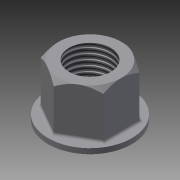
# Autodesk Inventor part: 13_17
Saved by Autodesk Inventor 2015 (Build 190159000, 159)
## iProperties
Created: 2015-04-06
Part Number: 13_17
Material: Generic
Document SubType Name: Modeling
Designer: WASHHSST
Density: 1 g/cm^3
Appearance: Default
Author: WASHHSST
Autodesk Inventor part; units mm, degrees
ref_plane "YZ Plane" through (0, 0, 0) normal (1, 0, 0) x (0, 1, 0)
ref_plane "XZ Plane" through (0, 0, 0) normal (0, 1, 0) x (-1, 0, 0)
ref_plane "XY Plane" through (0, 0, 0) normal (0, 0, 1) x (1, 0, 0)
sketch "Sketch1" plane through (0, 0, 0) normal (0, 1, 0) x (-1, 0, 0)
  circle A0 centre (0, 0) radius 25.4
  dimension "d0" = 50.8
  constraints: 1 centre point, 1 coincident
  measures "d0" diameter of A0
extrude "Extrusion1" add sketch "Sketch1" along normal blind 3.175
sketch "Sketch2" plane through (0, 3.175, 0) normal (0, 1, 0) x (1, 0, 0)
  circle A0 centre (0, 0) radius 19.05
  line L0 (-19.05, -10.9985) -> (-19.05, 10.9985)
  line L1 (-19.05, 10.9985) -> (0, 21.997)
  line L2 (0, 21.997) -> (19.05, 10.9985)
  line L3 (19.05, 10.9985) -> (19.05, -10.9985)
  line L4 (19.05, -10.9985) -> (0, -21.997)
  line L5 (0, -21.997) -> (-19.05, -10.9985)
  point P0 (-9.525, -16.4978)
  dimension "d3" = 38.1
  constraints: 12 end point, 2 coincident, 1 midpoint, 1 vertical, 16 other
extrude "Extrusion2" add sketch "Sketch2" along normal blind 28.575
sketch "Sketch3" plane through (0, 31.75, 0) normal (0, 1, 0) x (1, 0, 0)
  circle A0 centre (0, 0) radius 12.7
  dimension "d7" = 25.4
  constraints: 1 centre point, 1 coincident
  measures "d7" diameter of A0
extrude "Extrusion3" cut sketch "Sketch3" against normal through all
thread "Thread1" size "1-8 UNC" class "2B" standard "ANSI Unified Screw Threads" full length
sketch "Sketch6" plane through (0, 31.75, 0) normal (0, 1, 0) x (1, 0, 0)
  circle A0 centre (0, 0) radius 19.05
  line L0 (-19.05, -10.9985) -> (0, -21.997) projected
  constraints: 1 centre point, 1 coincident, 1 tangent
extrude "Extrusion5" cut sketch "Sketch6" against normal through all draft 45 keep common part
fillet "Fillet2" radius 1.524 6 edges at (-19.05, 3.175, 0) (-9.525, 3.175, 16.4978) (9.525, 3.175, 16.4978) (-9.525, 3.175, -16.4978) (9.525, 3.175, -16.4978) (19.05, 3.175, 0)
body "Solid1"
